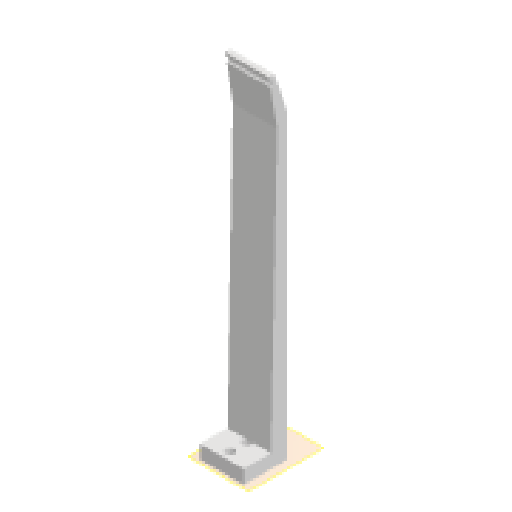
# Autodesk Inventor part: OT2-Gripper_finger
Saved by Autodesk Inventor 2024.1 (Build 281209000, 209)
## iProperties
Created: 2024-09-05
Part Number: OT2-Gripper_finger
Material: Generisch
Document SubType Name: Modeling
Designer: diederichbenedict
Density: 1 g/cm^3
Appearance: Vorgabe
Author: diederichbenedict
Autodesk Inventor part; units mm, degrees
ref_plane "YZ Plane" through (0, 0, 0) normal (1, 0, 0) x (0, 1, 0)
ref_plane "XZ Plane" through (0, 0, 0) normal (0, 1, 0) x (-1, 0, 0)
ref_plane "XY Plane" through (0, 0, 0) normal (0, 0, 1) x (1, 0, 0)
ref_plane "Arbeitsebene1" through (0, 10.2818, 0) normal (0, 0, 1) x (1, 0, 0)
sketch "Skizze1" plane through (0, 10.2818, 0) normal (0, 0, 1) x (1, 0, 0)
  circle A0 centre (10, 10.7182) radius 1.4 projected
  circle A1 centre (10, 4.7182) radius 1.4 projected
  circle A2 centre (10, -1.2818) radius 1.4 projected
  circle A3 centre (10, -7.2818) radius 1.4 projected
  line L0 (0, 12.7182) -> (2, 14.7182) projected
  line L1 (0, -8.2818) -> (0, 12.7182) projected
  line L2 (2, -10.2818) -> (0, -8.2818) projected
  line L3 (2, -10.2818) -> (18, -10.2818) projected
  line L4 (20, -8.2818) -> (18, -10.2818) projected
  line L5 (20, -8.2818) -> (20, 12.7182) projected
  line L6 (18, 14.7182) -> (20, 12.7182) projected
  line L7 (2, 14.7182) -> (18, 14.7182) projected
  line L8 (18, -10.2818) -> (2, -10.2818)
  line L9 (2, -10.2818) -> (2, 5.7182)
  line L10 (2, 5.7182) -> (18, 5.7182)
  line L11 (18, 5.7182) -> (18, -10.2818)
  circle A4 centre (10, -1.2818) radius 1.6
  circle A5 centre (10, -7.2818) radius 1.6
  point P0 (0, -10.2818)
  point P1 (2, -10.2818)
  dimension "d0" = 16
  dimension "d1" = 3.2
  dimension "d2" = 3.2
  constraints: 8 end point, 2 centre point, 2 coincident, 2 parallel, 1 horizontal, 1 perpendicular
  measures "d0" distance of L8.end L9.end
  measures "d1" diameter of A4
  measures "d2" diameter of A5
extrude "Extrusion1" add sketch "Skizze1" along normal blind 5 contours A1 L10 | A1 L10 L11 L3 L9 picked at (10.1558, 4.945)
sketch "Skizze2" plane through (18, 0, 0) normal (1, 0, 0) x (0, 0, -1)
  line L0 (0, 0) -> (0, 16) projected
  line L1 (0, 16) -> (-5, 16) projected
  line L2 (-5, 0) -> (-5, 16) projected
  line L3 (0, 0) -> (-5, 0) projected
  line L4 (-5, 16) -> (100, 16) construction
  line L5 (-103.3677, 42.3666) -> (-123.2187, 31.877)
  line L6 (-123.2187, 31.877) -> (-123.0578, 28.8814)
  line L7 (-123.0578, 28.8814) -> (-105.1383, 35)
  line L8 (-5, 10) -> (-85, 10)
  line L9 (-85, 10) -> (-105.1383, 35)
  line L10 (-5, 16) -> (-82.1287, 16)
  line L11 (-82.1287, 16) -> (-103.3677, 42.3666)
  point P0 (0, 0)
  point P1 (-123.1383, 30.3792)
  dimension "d8" = 3
  dimension "d9" = 6
  dimension "d15" = 80
  dimension "d16" = 6
  dimension "d17" = 9
  dimension "d18" = 110
  dimension "d19" = 18
  dimension "d20" = 25
  constraints: 16 end point, 3 horizontal, 1 midpoint, 1 parallel, 1 point on line
  measures "d8" distance of L5.end L6.end
  measures "d9" distance of L8.start L1.end
  measures "d15" distance of L8.start L8.end
  measures "d16" distance between parallel lines of L9 L11
  measures "d17" angle of L7 L5
  measures "d18" angle of L9 L7
  measures "d19" horizontal distance of point (-123.138, 30.379) L7.end
  measures "d20" vertical distance of L8.end L7.end
extrude "Extrusion2" add sketch "Skizze2" against normal up to surface (16 mm away) contours L2 L8 L9 L7 L6 L5 L11 L10
sketch "Skizze3" plane through (18, 0, 0) normal (1, 0, 0) x (0, 0, -1)
  line L0 (0, 0) -> (0, 16) projected
  line L1 (0, 16) -> (-82.1287, 16) projected
  line L2 (-103.3677, 42.3666) -> (-123.2187, 31.877) projected
  line L3 (-123.2187, 31.877) -> (-123.0578, 28.8814) projected
  line L4 (-123.0578, 28.8814) -> (-105.1383, 35) projected
  line L5 (-5, 0) -> (-5, 10) projected
  line L6 (0, 0) -> (-5, 0) projected
  circle A0 centre (-120.723, 29.6786) radius 1
  line L7 (-82.1287, 16) -> (-103.3677, 42.3666) projected
  line L8 (-105.1383, 35) -> (-85, 10) projected
  line L9 (-85, 10) -> (-5, 10) projected
  point P0 (0, 0)
  point P1 (-119.7766, 30.0017)
  point P2 (-121.6693, 29.3555)
  dimension "d12" = 2
  constraints: 1 centre point, 1 point on line
  measures "d12" diameter of A0
extrude "Extrusion3" cut sketch "Skizze3" against normal through all contours L4 A0 picked at (-121.0524, 29.7298)
